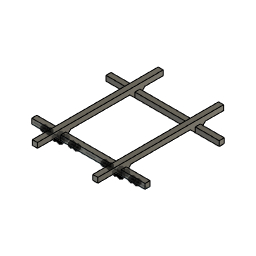
底架（仿） (Autodesk Fusion 360 design; units mm, degrees)
Autodesk Fusion 360 part; units mm, degrees
sketch "草图1" plane through (0, 0, 0) normal (0, 0, 1) x (1, 0, 0)
  line L0 (110, -137.5) -> (-110, -137.5)
  line L1 (-110, -137.5) -> (-110, 137.5)
  line L2 (-110, 137.5) -> (110, 137.5)
  line L3 (110, 137.5) -> (110, -137.5)
  line L4 (110, -137.5) -> (-110, 137.5) construction
  line L5 (-110, -137.5) -> (110, 137.5) construction
  line L6 (130, -157.5) -> (-130, -157.5)
  line L7 (-130, -157.5) -> (-130, 157.5)
  line L8 (-130, 157.5) -> (130, 157.5)
  line L9 (130, 157.5) -> (130, -157.5)
  line L10 (130, -157.5) -> (-130, 157.5) construction
  line L11 (-130, -157.5) -> (130, 157.5) construction
  line L12 (110, 137.5) -> (225, 137.5)
  line L13 (225, 137.5) -> (-225, 137.5)
  line L14 (0, 0) -> (0, 157.5) construction
  line L15 (0, 0) -> (0, -157.5) construction
  line L16 (-110, 137.5) -> (-110, 250)
  line L17 (-110, 250) -> (-110, -250)
  line L18 (0, 0) -> (-130, 0) construction
  line L19 (-225, 250) -> (225, 250)
  line L20 (225, 250) -> (225, -250)
  line L21 (225, -250) -> (-225, -250)
  line L22 (-225, -250) -> (-225, 250)
  line L23 (-225, 250) -> (225, -250) construction
  line L24 (225, 250) -> (-225, -250) construction
  line L25 (-130, 250) -> (-130, -250)
  line L26 (225, -157.5) -> (-225, -157.5)
  line L27 (-225, -137.5) -> (225, -137.5)
  line L28 (110, 250) -> (110, -250)
  line L29 (130, -250) -> (130, 250)
  line L30 (225, 157.5) -> (-225, 157.5)
  point P0 (-110, 0)
  dimension "d1" = 220
  dimension "d2" = 275
  dimension "d3" = 20
  dimension "d4" = 20
  dimension "d5" = 450
  dimension "d6" = 95
  dimension "d7" = 95
  dimension "d8" = 500
  dimension "d9" = 92.5
  dimension "d15" = 450
  dimension "d16" = 500
  constraint horizontal L0
  constraint perpendicular L0 L1
  constraint parallel L0 L2
  constraint parallel L1 L3
  constraint coincident L4 L14.start
  constraint coincident L5 L14.start
  constraint coincident L14.start L15.start
  constraint horizontal L6
  constraint perpendicular L6 L7
  constraint parallel L6 L8
  constraint parallel L7 L9
  constraint coincident L10 L14.start
  constraint coincident L11 L14.start
  constraint perpendicular L3 L12
  constraint perpendicular L7 L13
  constraint midpoint L8 L14.end
  constraint midpoint L6 L15.end
  constraint symmetric L12.end L13.end L14
  constraint perpendicular L13 L16
  constraint perpendicular L6 L17
  constraint midpoint L7 L18.end
  constraint coincident L18 P0
  constraint symmetric L16.end L17.end L18
  constraint horizontal L19
  constraint perpendicular L19 L20
  constraint parallel L19 L21
  constraint parallel L20 L22
  constraint coincident L23 L14.start
  constraint coincident L24 L14.start
  constraint coincident L13.end L22
  constraint coincident L16.end L19
  constraint coincident L19 L25.start
  constraint coincident L21 L25.end
  constraint perpendicular L21 L25
  constraint coincident L20 L26.start
  constraint coincident L22 L26.end
  constraint perpendicular L22 L26
  constraint coincident L22 L27.start
  constraint coincident L20 L27.end
  constraint perpendicular L20 L27
  constraint coincident L19 L28.start
  constraint coincident L21 L28.end
  constraint perpendicular L21 L28
  constraint coincident L21 L29.start
  constraint coincident L19 L29.end
  constraint perpendicular L19 L29
  constraint coincident L20 L30.start
  constraint coincident L22 L30.end
  constraint perpendicular L22 L30
  measures "d1" distance of L1.end L2.end
  measures "d2" distance of L0.end L1.end
  measures "d3" distance of L3 L9
  measures "d4" distance of L2 L8
  measures "d5" distance of L12.end L13.end
  measures "d6" distance of L9 L12.end
  measures "d7" distance of L7 L13.end
  measures "d8" distance of L16.end L17.end
  measures "d9" distance of L8 L16.end
  measures "d15" distance of L20 L22
  measures "d16" distance of L19 L21
extrude "拉伸1" add sketch "草图1" along normal blind 20 contours L3 L9 L12 L13 L27 L28 L29 | L6 L9 L26 L27 L28 L29 | L1 L7 L13 L17 L25 L27 | L6 L7 L17 L25 L26 L27 | L8 L9 L12 L13 L28 L29 L30 | L6 L21 L26 L28 L29 | L7 L8 L13 L16 L17 L25 L30 | L6 L17 L21 L25 L26 | L8 L19 L28 L29 L30 | L8 L16 L17 L19 L25 L30 makes body 1 at (-110, 83.3333, 6.6667) makes body 2 at (130, 83.3333, 6.6667)
extrude "拉伸2" add sketch "草图1" against normal blind 20 contours L0 L6 L17 L26 L27 L28 | L6 L9 L26 L27 L28 L29 | L6 L7 L17 L25 L26 L27 | L8 L9 L12 L13 L28 L29 L30 | L2 L8 L13 L16 L17 L28 L30 | L9 L20 L26 L27 L29 | L7 L8 L13 L16 L17 L25 L30 | L7 L22 L25 L26 L27 | L9 L12 L13 L20 L29 L30 | L7 L13 L22 L25 L30 bodies 1 2
chamfer "倒角1" distance 20 angle 45 8 edges at (-120, -157.5, 0) (120, -157.5, 0) (-120, 137.5, 0) (120, 137.5, 0) (-120, -137.5, 0) (-120, 157.5, 0) (120, 157.5, 0) (120, -137.5, 0) on bodies 1
sketch "草图2" plane through (0, 0, -20) normal (0, 0, -1) x (1, 0, 0)
  line L0 (-225, 157.5) -> (-225, 137.5)
  line L1 (-225, 137.5) -> (-130, 137.5)
  line L2 (-130, 137.5) -> (-110, 137.5)
  line L3 (-110, 137.5) -> (110, 137.5)
  line L4 (110, 137.5) -> (130, 137.5)
  line L5 (130, 137.5) -> (225, 137.5)
  line L6 (225, 137.5) -> (225, 157.5)
  line L7 (225, 157.5) -> (130, 157.5)
  line L8 (130, 157.5) -> (110, 157.5)
  line L9 (110, 157.5) -> (-110, 157.5)
  line L10 (-110, 157.5) -> (-130, 157.5)
  line L11 (-130, 157.5) -> (-225, 157.5)
  line L12 (-130, 157.5) -> (-130, 137.5) construction
  line L13 (-110, 157.5) -> (-110, 137.5) construction
  line L14 (110, 157.5) -> (110, 137.5) construction
  line L15 (130, 157.5) -> (130, 137.5) construction
  line L16 (-225, 147.5) -> (225, 147.5) construction
  circle A0 centre (-185.15, 147.5) radius 2.65
  circle A1 centre (-164.85, 147.5) radius 2.65
  circle A2 centre (164.85, 147.5) radius 2.65
  circle A3 centre (185.15, 147.5) radius 2.65
  circle A4 centre (-75.15, 147.5) radius 2.65
  circle A5 centre (-54.85, 147.5) radius 2.65
  circle A6 centre (54.85, 147.5) radius 2.65
  circle A7 centre (75.15, 147.5) radius 2.65
  point P0 (-185.15, 147.5)
  point P1 (-164.85, 147.5)
  point P2 (164.85, 147.5)
  point P3 (185.15, 147.5)
  point P4 (-75.15, 147.5)
  point P5 (-54.85, 147.5)
  point P6 (75.15, 147.5)
  point P7 (54.85, 147.5)
  dimension "d17" = 55.15
  dimension "d18" = 55.15
  dimension "d19" = 20.3
  dimension "d20" = 20.3
  dimension "d21" = 5.3
  dimension "d22" = 5.3
  dimension "d23" = 5.3
  dimension "d24" = 5.3
  dimension "d25" = 55.15
  dimension "d26" = 55.15
  dimension "d27" = 20.3
  dimension "d28" = 20.3
  dimension "d29" = 5.3
  dimension "d30" = 5.3
  dimension "d31" = 5.3
  dimension "d32" = 5.3
  constraint coincident L10.end L11.start
  constraint coincident L1.end L2.start
  constraint coincident L9.end L10.start
  constraint coincident L2.end L3.start
  constraint coincident L8.end L9.start
  constraint coincident L3.end L4.start
  constraint coincident L7.end L8.start
  constraint coincident L4.end L5.start
  constraint midpoint L0 L16.start
  constraint midpoint L6 L16.end
  constraint coincident L16 P0
  constraint coincident L16 P1
  constraint coincident L16 P2
  constraint coincident L16 P3
  constraint coincident P0 A0.centre
  constraint coincident P1 A1.centre
  constraint coincident P2 A2.centre
  constraint coincident P3 A3.centre
  constraint coincident L16 P4
  constraint coincident L16 P5
  constraint coincident L16 P6
  constraint coincident L16 P7
  constraint coincident P4 A4.centre
  constraint coincident P5 A5.centre
  constraint coincident P7 A6.centre
  constraint coincident P6 A7.centre
  measures "d17" distance of L12 P0
  measures "d18" distance of L15 P3
  measures "d19" distance of P0 P1
  measures "d20" distance of P2 P3
  measures "d21" diameter of A0
  measures "d22" diameter of A1
  measures "d23" diameter of A2
  measures "d24" diameter of A3
  measures "d25" horizontal distance of L2.end P5
  measures "d26" distance of L14 P7
  measures "d27" distance of P4 P5
  measures "d28" distance of P6 P7
  measures "d29" diameter of A4
  measures "d30" diameter of A5
  measures "d31" diameter of A6
  measures "d32" diameter of A7
extrude "拉伸3" cut sketch "草图2" against normal blind 10 contours A0 | A1 | A2 | A3 | A4 | A5 | A6 | A7 bodies 1
sketch "草图3" plane through (0, 0, -20) normal (0, 0, -1) x (1, 0, 0)
  line L0 (225, -157.5) -> (225, -137.5)
  line L1 (225, -137.5) -> (130, -137.5)
  line L2 (130, -137.5) -> (110, -137.5)
  line L3 (110, -137.5) -> (-110, -137.5)
  line L4 (-110, -137.5) -> (-130, -137.5)
  line L5 (-130, -137.5) -> (-225, -137.5)
  line L6 (-225, -137.5) -> (-225, -157.5)
  line L7 (-225, -157.5) -> (-130, -157.5)
  line L8 (-130, -157.5) -> (-110, -157.5)
  line L9 (-110, -157.5) -> (110, -157.5)
  line L10 (110, -157.5) -> (130, -157.5)
  line L11 (130, -157.5) -> (225, -157.5)
  line L12 (-130, -137.5) -> (-130, -157.5)
  line L13 (-110, -137.5) -> (-110, -157.5)
  line L14 (110, -137.5) -> (110, -157.5)
  line L15 (130, -137.5) -> (130, -157.5)
  line L16 (225, -147.5) -> (-225, -147.5) construction
  circle A0 centre (-185.15, -147.5) radius 2.65
  circle A1 centre (-164.85, -147.5) radius 2.65
  circle A2 centre (-75.15, -147.5) radius 2.65
  circle A3 centre (-54.85, -147.5) radius 2.65
  circle A4 centre (54.85, -147.5) radius 2.65
  circle A5 centre (75.15, -147.5) radius 2.65
  circle A6 centre (164.85, -147.5) radius 2.65
  circle A7 centre (185.15, -147.5) radius 2.65
  point P0 (-164.85, -147.5)
  point P1 (-185.15, -147.5)
  point P2 (-75.15, -147.5)
  point P3 (-54.85, -147.5)
  point P4 (54.85, -147.5)
  point P5 (75.15, -147.5)
  point P6 (164.85, -147.5)
  point P7 (185.15, -147.5)
  dimension "d35" = 5.3
  dimension "d36" = 5.3
  dimension "d37" = 5.3
  dimension "d38" = 5.3
  dimension "d39" = 5.3
  dimension "d40" = 5.3
  dimension "d41" = 5.3
  dimension "d42" = 5.3
  dimension "d43" = 55.15
  dimension "d44" = 55.15
  dimension "d45" = 55.15
  dimension "d46" = 55.15
  dimension "d47" = 20.3
  dimension "d48" = 20.3
  dimension "d49" = 20.3
  dimension "d50" = 20.3
  constraint coincident L4.end L5.start
  constraint coincident L7.end L8.start
  constraint coincident L3.end L4.start
  constraint coincident L8.end L9.start
  constraint coincident L2.end L3.start
  constraint coincident L9.end L10.start
  constraint coincident L1.end L2.start
  constraint coincident L10.end L11.start
  constraint midpoint L0 L16.start
  constraint midpoint L6 L16.end
  constraint coincident L16 P0
  constraint coincident L16 P1
  constraint coincident L16 P2
  constraint coincident L16 P3
  constraint coincident L16 P4
  constraint coincident L16 P5
  constraint coincident L16 P6
  constraint coincident L16 P7
  constraint coincident P1 A0.centre
  constraint coincident P0 A1.centre
  constraint coincident P2 A2.centre
  constraint coincident P3 A3.centre
  constraint coincident P4 A4.centre
  constraint coincident P5 A5.centre
  constraint coincident P6 A6.centre
  constraint coincident P7 A7.centre
  measures "d35" diameter of A0
  measures "d36" diameter of A1
  measures "d37" diameter of A2
  measures "d38" diameter of A3
  measures "d39" diameter of A4
  measures "d40" diameter of A5
  measures "d41" diameter of A6
  measures "d42" diameter of A7
  measures "d43" distance of L12 P1
  measures "d44" distance of L13 P3
  measures "d45" distance of L14 P4
  measures "d46" distance of L15 P7
  measures "d47" distance of P6 P7
  measures "d48" distance of P4 P5
  measures "d49" distance of P2 P3
  measures "d50" distance of P0 P1
extrude "拉伸4" cut sketch "草图2" sketch "草图3" against normal blind 5 contours A0 | A1 | A2 | A3 | A4 | A5 | A6 | A7 of sketch 2 contours A0 | A1 | A2 | A3 | A4 | A5 | A6 | A7 bodies 1
